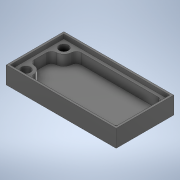
# Autodesk Inventor part: BottomCover
Saved by Autodesk Inventor 2020 (Build 240168000, 168)
## iProperties
Created: 2021-11-07
Part Number: BottomCover
Material: アセタール樹脂、黒
Document SubType Name: Modeling
Designer: Masato Kubotera
Density: 1.425 g/cm^3
Appearance: 滑らか - 黒
Author: Masato Kubotera
## iProperties of the stored document _3D プリント.ipt
Created: 2021-11-07
Part Number: _3D プリント
Material: 一般
Document SubType Name: Modeling
Designer: Masato Kubotera
Density: 1 g/cm^3
Appearance: 既定
Author: Masato Kubotera
Autodesk Inventor part; units mm, degrees
ref_plane "YZ Plane" through (0, 0, 0) normal (1, 0, 0) x (0, 1, 0)
ref_plane "XZ Plane" through (0, 0, 0) normal (0, 1, 0) x (-1, 0, 0)
ref_plane "XY Plane" through (0, 0, 0) normal (0, 0, 1) x (1, 0, 0)
sketch "スケッチ1" plane through (0, 0, 0) normal (0, 0, 1) x (1, 0, 0)
  line L0 (-10, 20) -> (10, 20) construction
  line L1 (10, 20) -> (10, -20) construction
  line L2 (10, -20) -> (-10, -20) construction
  line L3 (-10, -20) -> (-10, 20) construction
  line L4 (-10, 20) -> (10, -20) construction
  line L5 (10, 20) -> (-10, -20) construction
  circle A0 centre (-7.25, 17.25) radius 1.75
  line L6 (0, 20) -> (0, -20) construction
  circle A1 centre (7.25, 17.25) radius 1.75
  line L7 (9, -19) -> (-9, -19)
  line L8 (-9, -19) -> (-9, 14.8133)
  line L9 (-9, 19) -> (-4.8133, 19) construction
  line L10 (9, 19) -> (9, 14.8133) construction
  line L11 (9, -19) -> (-9, 19) construction
  line L12 (-9, -19) -> (9, 19) construction
  arc A2 (-9, 14.8133) -> (-4.8133, 19) centre (-7.25, 17.25) ccw
  line L13 (-4.8133, 19) -> (4.8133, 19)
  line L14 (-9, 14.8133) -> (-9, 19) construction
  arc A3 (4.8133, 19) -> (9, 14.8133) centre (7.25, 17.25) ccw
  line L15 (4.8133, 19) -> (9, 19) construction
  line L16 (9, 14.8133) -> (9, -19)
  line L17 (-11, 21) -> (11, 21)
  line L18 (11, 21) -> (11, -21)
  line L19 (11, -21) -> (-11, -21)
  line L20 (-11, -21) -> (-11, 21)
  line L21 (-11, 21) -> (11, -21) construction
  line L22 (11, 21) -> (-11, -21) construction
  line L23 (10.25, -20.25) -> (-10.25, -20.25)
  line L24 (-10.25, -20.25) -> (-10.25, 20.25)
  line L25 (-10.25, 20.25) -> (10.25, 20.25)
  line L26 (10.25, 20.25) -> (10.25, -20.25)
  line L27 (10.25, -20.25) -> (-10.25, 20.25) construction
  line L28 (-10.25, -20.25) -> (10.25, 20.25) construction
  point P0 (0, 0)
  point P1 (0, 0)
  dimension "d0" = 20
  dimension "d1" = 40
  dimension "d2" = 3.5
  dimension "d3" = 2.75
  dimension "d4" = 2.75
  dimension "d5" = 1
  dimension "d6" = 1
  dimension "d7" = 3
  dimension "d13" = 1
  dimension "d14" = 1
  dimension "d15" = 0.25
  dimension "d16" = 0.25
  constraints: 58 end point, 13 parallel, 12 midpoint, 5 perpendicular, 4 centre point, 4 horizontal, 4 point on circle, 4 symmetric about line, 1 coincident, 2 other
  measures "d0" distance of L1.end L2.end
  measures "d1" distance of L0.end L1.end
  measures "d2" diameter of A0
  measures "d3" distance from line of L3 A0.centre
  measures "d4" horizontal distance of L0.start A0.centre
  measures "d5" distance between parallel lines of L0 L9
  measures "d6" distance between parallel lines of L3 L8
  measures "d7" radius of A2
  measures "d13" distance between parallel lines of L17 L0
  measures "d14" distance between parallel lines of L20 L3
  measures "d15" distance between parallel lines of L0 L25
  measures "d16" distance between parallel lines of L24 L3
extrude "押し出し1" add sketch "スケッチ1" along normal blind 6.6 contours L17 L18 L19 L20
extrude "押し出し2" add sketch "スケッチ1" along normal blind 1 contours L7 L8 A2 L13 A3 L16 | L23 L24 L25 L26
extrude "押し出し3" add sketch "スケッチ1" along normal blind 5 contours L17 L18 L19 L20 | L23 L24 L25 L26
fillet "フィレット1" radius 2 6 edges at (-9, 14.8133, 3) (-4.8133, 19, 3) (4.8133, 19, 3) (9, 14.8133, 3) (-9, -19, 3) (9, -19, 3)
equation "\"d4\" = d3"
equation "\"d6\" = d5"
equation "\"d14\" = d5"
